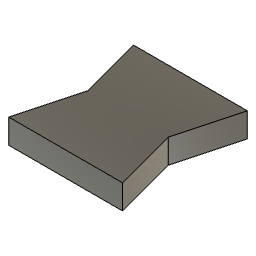
tile_lock v3 (Autodesk Fusion 360 design; units mm, degrees)
Autodesk Fusion 360 part; units mm, degrees
sketch "Sketch1" plane through (0, 0, 0) normal (0, 0, 1) x (1, 0, 0)
  line L0 (0, 0) -> (5, 0) construction
  line L1 (5, 0) -> (7.0706, 7.7274) construction
  line L2 (5, 0) -> (13, 0) construction
  line L3 (5, 0) -> (7.0706, -7.7274) construction
  line L4 (5, 0) -> (13, 0) construction
  line L5 (0, 0) -> (-5, 0) construction
  line L6 (-5, 0) -> (-7.0706, 7.7274) construction
  line L7 (-5, 0) -> (0, 0) construction
  line L8 (-5, 0) -> (-7.0706, -7.7274) construction
  line L9 (-5, 0) -> (0, 0) construction
  line L10 (-7.0706, -7.7274) -> (7.0706, -7.7274) construction
  line L11 (-7.0706, 7.7274) -> (7.0706, 7.7274) construction
  line L12 (0, 0) -> (4.95, 0) construction
  line L13 (4.95, 0) -> (7.0076, 7.6791)
  line L14 (4.95, 0) -> (12.8, 0) construction
  line L15 (4.95, 0) -> (7.0076, -7.6791)
  line L16 (4.95, 0) -> (12.8, 0) construction
  line L17 (0, 0) -> (-4.95, 0) construction
  line L18 (-4.95, 0) -> (-7.0076, 7.6791)
  line L19 (-4.95, 0) -> (3, 0) construction
  line L20 (-7.0076, 7.6791) -> (7.0076, 7.6791)
  line L21 (-4.95, 0) -> (-7.0076, -7.6791)
  line L22 (-7.0076, -7.6791) -> (7.0076, -7.6791)
  dimension "d1" = 5
  dimension "d2" = 75
  dimension "d3" = 8
  dimension "d4" = 75
  dimension "d5" = 8
  dimension "d6" = 5
  dimension "d7" = 105
  dimension "d8" = 8
  dimension "d9" = 105
  dimension "d10" = 8
  dimension "d11" = 4.95
  dimension "d12" = 75
  dimension "d13" = 7.95
  dimension "d14" = 75
  dimension "d15" = 7.95
  dimension "d16" = 4.95
  dimension "d17" = 105
  dimension "d18" = 7.95
  dimension "d19" = 75
  dimension "d20" = 7.95
  constraint coincident L0.start L5.start
  constraint horizontal L0
  constraint horizontal L2
  constraint horizontal L4
  constraint horizontal L5
  constraint horizontal L7
  constraint horizontal L9
  constraint horizontal L12
  constraint horizontal L14
  constraint horizontal L16
  constraint parallel L7 L17
  constraint horizontal L19
  measures "d1" distance of L0.start L0.end
  measures "d2" angle of L1 L2
  measures "d3" distance of L0.end L1.end
  measures "d4" angle of L3 L4
  measures "d5" distance of L0.end L3.end
  measures "d6" distance of L0.start L5.end
  measures "d7" angle of L6 L7
  measures "d8" distance of L5.end L6.end
  measures "d9" angle of L8 L9
  measures "d10" distance of L5.end L8.end
  measures "d11" distance of L0.start L12.end
  measures "d12" angle of L13 L14
  measures "d13" distance of L12.end L13.end
  measures "d14" angle of L15 L16
  measures "d15" distance of L12.end L15.end
  measures "d16" distance of L0.start L17.end
  measures "d17" angle of L18 L19
  measures "d18" distance of L17.end L18.end
  measures "d19" angle of L20 L21
  measures "d20" distance of L17.end L21.end
extrude "Extrude1" add sketch "Sketch1" along normal blind 3
